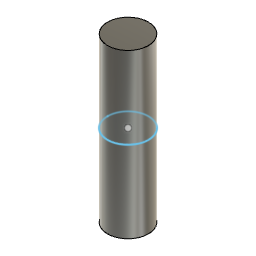
Pilon 3 (Autodesk Fusion 360 design; units mm, degrees)
Autodesk Fusion 360 part; units mm, degrees
sketch "sketch 312" plane through (0, 0, 15) normal (0, 0, 1) x (-1, 0, 0)
  circle A0 centre (-87.5, -5) radius 2.5
  circle A1 centre (-87.5, -5) radius 2.5
extrude "Extrude1" add sketch "sketch 312" along normal blind -10 and the other way blind -5
extrude "Extrude2" add 1 faces at (87.8045, 5.7757, 20) along direction (0, 0, 1) blind 5
